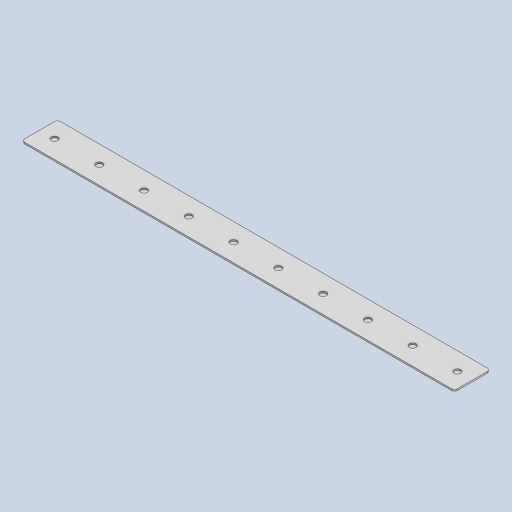
# Autodesk Inventor part: sheet
Saved by Autodesk Inventor 2023 (Build 270158000, 158)
## iProperties
Created: 2024-12-14
Part Number: sheet
Material: Generic
Document SubType Name: Modeling
Designer: kiyo
Density: 1 g/cm^3
Appearance: Default
Author: kiyo
Autodesk Inventor part; units mm, degrees
ref_plane "YZ Plane" through (0, 0, 0) normal (1, 0, 0) x (0, 1, 0)
ref_plane "XZ Plane" through (0, 0, 0) normal (0, 1, 0) x (-1, 0, 0)
ref_plane "XY Plane" through (0, 0, 0) normal (0, 0, 1) x (1, 0, 0)
sketch "スケッチ1" plane through (0, 0, 0) normal (0, 0, 1) x (1, 0, 0)
  line L0 (0, 0) -> (-12, 0)
  line L1 (-12, 0) -> (-12, -145)
  line L2 (-12, -145) -> (0, -145)
  line L3 (0, -145) -> (0, 0)
  circle A0 centre (-6, -140) radius 1.1
  circle A1 centre (-6, -125) radius 1.1
  circle A2 centre (-6, -110) radius 1.1
  circle A3 centre (-6, -95) radius 1.1
  circle A4 centre (-6, -80) radius 1.1
  circle A5 centre (-6, -65) radius 1.1
  circle A6 centre (-6, -50) radius 1.1
  circle A7 centre (-6, -35) radius 1.1
  circle A8 centre (-6, -20) radius 1.1
  circle A9 centre (-6, -5) radius 1.1
  dimension "d0" = 145
  dimension "d1" = 12
  dimension "d2" = 2.2
  dimension "d3" = 5
  dimension "d4" = 6
  dimension "d7" = 15
  constraints: 10 centre point, 8 end point, 2 parallel, 1 horizontal, 1 perpendicular, 1 vertical, 18 other
  measures "d0" distance of L0.end L1.end
  measures "d1" distance of L1.end L2.end
  measures "d2" diameter of A0
  measures "d3" distance from line of L2 A0.centre
  measures "d4" distance from line of L1 A0.centre
  measures "d7" distance of A0.centre A1.centre
extrude "押し出し1" add sketch "スケッチ1" along normal blind 0.5
fillet "フィレット1" radius 1 4 edges at (-12, -145, 0.25) (0, -145, 0.25) (0, 0, 0.25) (-12, 0, 0.25)
equation "\"d4\" = 0.5 * d1"
